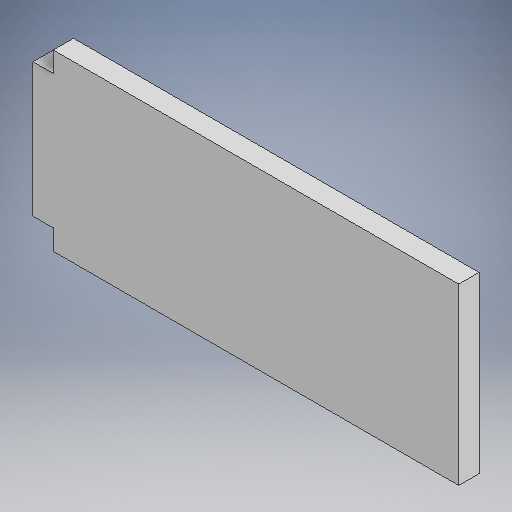
# Autodesk Inventor part: floor1
Saved by Autodesk Inventor 2025.3 (Build 293356000, 356)
## iProperties
Created: 2026-04-15
Part Number: floor1
Material: Generic
Document SubType Name: Modeling
Designer: user
Density: 1 g/cm^3
Appearance: Default
Author: user
Autodesk Inventor part; units mm, degrees
ref_plane "YZ Plane" through (0, 0, 0) normal (1, 0, 0) x (0, 1, 0)
ref_plane "XZ Plane" through (0, 0, 0) normal (0, 1, 0) x (-1, 0, 0)
ref_plane "XY Plane" through (0, 0, 0) normal (0, 0, 1) x (1, 0, 0)
sketch "Sketch1" plane through (0, 0, 0) normal (0, 0, 1) x (1, 0, 0)
  line L0 (-62.0787, -12.8855) -> (-42.0787, -12.8855) construction
  line L1 (-42.0787, -12.8855) -> (-42.0787, 20.1145)
  line L2 (-42.0787, 20.1145) -> (-37.0787, 20.1145)
  line L3 (-37.0787, 20.1145) -> (-37.0787, 25.1145)
  line L4 (-37.0787, 25.1145) -> (62.9213, 25.1145)
  line L5 (-42.0787, -12.8855) -> (-37.0787, -12.8855)
  line L6 (62.9213, -17.8855) -> (-37.0787, -17.8855)
  line L7 (-37.0787, -17.8855) -> (-37.0787, -12.8855)
  line L8 (62.9213, 25.1145) -> (62.9213, -17.8855)
  point P0 (0, 0)
  dimension "d1" = 33
  dimension "d2" = 5
  dimension "d3" = 5
  dimension "d4" = 100
  dimension "d9" = 5
  constraints: 18 end point, 5 horizontal, 3 vertical, 1 parallel, 1 perpendicular
  measures "d1" distance of L0.end L2.start
  measures "d2" distance of L2.start L3.start
  measures "d3" distance of L3.start L3.end
  measures "d4" distance of L3.end L4.end
  measures "d9" distance of L7.start L5.end
extrude "Extrusion1" add sketch "Sketch1" along normal blind 5
body "Solid1"
